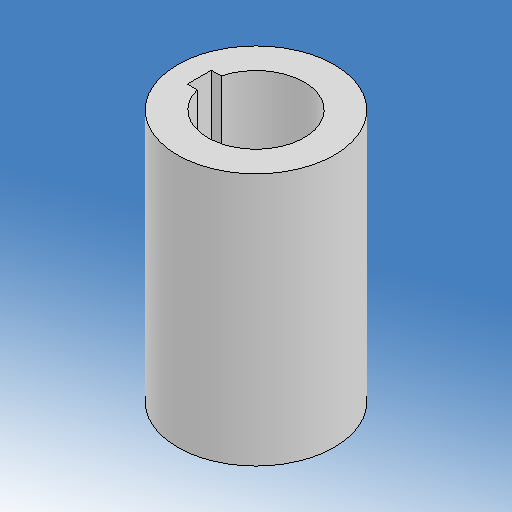
# Autodesk Inventor part: 8mmKeyedShaftLongSpacer_BevelToSpurShaft
Saved by Autodesk Inventor 2025 (Build 290162000, 162)
## iProperties
Created: 2024-06-12
Part Number: 8mmKeyedShaftLongSpacer_BevelToSpurShaft
Material: Generic
Document SubType Name: Modeling
Designer: seene
Density: 1 g/cm^3
Appearance: Default
Author: seene
Autodesk Inventor part; units mm, degrees
ref_plane "YZ Plane" through (0, 0, 0) normal (1, 0, 0) x (0, 1, 0)
ref_plane "XZ Plane" through (0, 0, 0) normal (0, 1, 0) x (-1, 0, 0)
ref_plane "XY Plane" through (0, 0, 0) normal (0, 0, 1) x (1, 0, 0)
sketch "Sketch1" plane through (0, 0, 0) normal (0, 1, 0) x (-1, 0, 0)
  circle A0 centre (0, 0) radius 4
  circle A1 centre (0, 0) radius 6.5
  line L0 (2.7, 1) -> (4.7, 1)
  line L1 (4.7, 1) -> (4.7, -1)
  line L2 (4.7, -1) -> (2.7, -1)
  line L3 (2.7, -1) -> (2.7, 1)
  line L4 (4.6972, 0) -> (0, 0) construction
  line L5 (3.7, 1) -> (3.7, -1) construction
  line L6 (4.7, 0) -> (0, 0) construction
  point P0 (3.873, -1)
  point P1 (3.873, 1)
  dimension "d0" = 8
  dimension "d1" = 2.5
  dimension "d2" = 2
  dimension "d3" = 2
  dimension "d6" = 2.7
  constraints: 14 end point, 3 horizontal, 3 midpoint, 2 centre point, 2 parallel, 1 coincident, 1 perpendicular
  measures "d0" diameter of A0
  measures "d1" radial gap between concentric circles of A0 A1
  measures "d2" distance between parallel lines of L3 L1
  measures "d3" distance of L2.end L0.start
  measures "d6" distance from line of point (0, 0) L3
extrude "Extrusion1" add sketch "Sketch1" along normal blind 21
body "Solid1"
